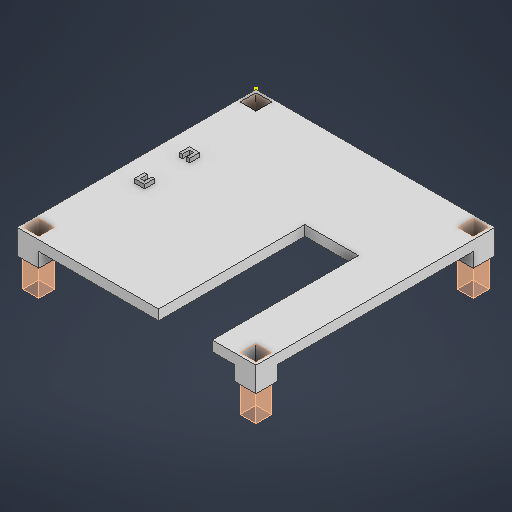
# Autodesk Inventor part: piano superiore
Saved by Autodesk Inventor 2026.2 (Build 302298000, 298)
## iProperties
Created: 2026-01-19
Part Number: piano superiore
Material: Generic
Document SubType Name: Modeling
Designer: ASUS
Density: 1 g/cm^3
Appearance: Default
Author: ASUS
Autodesk Inventor part; units mm, degrees
ref_plane "YZ Plane" through (0, 0, 0) normal (1, 0, 0) x (0, 1, 0)
ref_plane "XZ Plane" through (0, 0, 0) normal (0, 1, 0) x (-1, 0, 0)
ref_plane "XY Plane" through (0, 0, 0) normal (0, 0, 1) x (1, 0, 0)
sketch "Sketch1" plane through (0, 0, 0) normal (0, 1, 0) x (-1, 0, 0)
  line L0 (0, 0) -> (-165, 0)
  line L1 (-165, 0) -> (-165, 165)
  line L2 (-165, 165) -> (0, 165)
  line L3 (0, 165) -> (0, 0)
  line L4 (-165, 165) -> (-150, 165)
  line L5 (-165, 150) -> (-165, 165)
  line L6 (-163, 152) -> (-152, 152)
  line L7 (-152, 152) -> (-152, 163)
  line L8 (-152, 163) -> (-163, 163)
  line L9 (-163, 163) -> (-163, 152)
  line L10 (-2, 152) -> (-13, 152)
  line L11 (-13, 152) -> (-13, 163)
  line L12 (-13, 163) -> (-2, 163)
  line L13 (-2, 163) -> (-2, 152)
  line L14 (-163, 13) -> (-152, 13)
  line L15 (-152, 13) -> (-152, 2)
  line L16 (-152, 2) -> (-163, 2)
  line L17 (-163, 2) -> (-163, 13)
  line L18 (-2, 13) -> (-13, 13)
  line L19 (-13, 13) -> (-13, 2)
  line L20 (-13, 2) -> (-2, 2)
  line L21 (-2, 2) -> (-2, 13)
  line L22 (-150, 150) -> (-165, 150)
  line L23 (-165, 150) -> (-165, 165)
  line L24 (-165, 165) -> (-150, 165)
  line L25 (-150, 165) -> (-150, 150)
  line L26 (-150, 15) -> (-165, 15)
  line L27 (-165, 15) -> (-165, 0)
  line L28 (-165, 0) -> (-150, 0)
  line L29 (-150, 0) -> (-150, 15)
  line L30 (-15, 15) -> (0, 15)
  line L31 (0, 15) -> (0, 0)
  line L32 (0, 0) -> (-15, 0)
  line L33 (-15, 0) -> (-15, 15)
  line L34 (-15, 150) -> (0, 150)
  line L35 (0, 150) -> (0, 165)
  line L36 (0, 165) -> (-15, 165)
  line L37 (-15, 165) -> (-15, 150)
  line L38 (-165, 165) -> (-133.75, 165)
  line L39 (-133.75, 165) -> (-97.75, 165)
  line L40 (-97.75, 165) -> (-97.75, 64)
  line L41 (-97.75, 64) -> (-133.75, 64)
  line L42 (-133.75, 64) -> (-133.75, 165)
  point P0 (0, 15)
  dimension "d0" = 165
  dimension "d1" = 165
  dimension "d5" = 2
  dimension "d6" = 2
  dimension "d7" = 2
  dimension "d8" = 2
  dimension "d9" = 31.25
  dimension "d10" = 36
  dimension "d11" = 101
  constraints: 86 end point, 8 parallel, 4 perpendicular, 3 horizontal, 1 point on line, 13 other
  measures "d0" distance of L1.end L2.end
  measures "d1" distance of L0.end L1.end
  measures "d5" distance between parallel lines of L6 L22
  measures "d6" distance between parallel lines of L14 L26
  measures "d7" distance between parallel lines of L18 L30
  measures "d8" distance between parallel lines of L10 L34
  measures "d9" distance of L23.end L38.end
  measures "d10" distance of L40.end L41.end
  measures "d11" distance of L39.end L40.end
extrude "Extrusion1" add sketch "Sketch1" along normal blind 7 contours L0 L29 L26 L1 L22 L25 L2 L42 L41 L40 L37 L34 L3 L30 L33
sketch "Sketch2" plane through (0, 7, 0) normal (0, 1, 0) x (1, 0, 0)
  line L0 (15, -15) -> (0, -15) projected
  line L1 (15, -15) -> (0, -15)
  line L2 (0, -15) -> (0, 0)
  line L3 (0, 0) -> (15, 0)
  line L4 (15, 0) -> (15, -15)
  line L5 (150, -15) -> (150, 0) projected
  line L6 (150, -15) -> (165, -15)
  line L7 (165, -15) -> (165, 0)
  line L8 (165, 0) -> (150, 0)
  line L9 (150, 0) -> (150, -15)
  line L10 (150, -150) -> (165, -150) projected
  line L11 (150, -150) -> (165, -150)
  line L12 (165, -150) -> (165, -165)
  line L13 (165, -165) -> (150, -165)
  line L14 (150, -165) -> (150, -150)
  line L15 (15, -150) -> (0, -150)
  line L16 (0, -150) -> (0, -165)
  line L17 (0, -165) -> (15, -165)
  line L18 (15, -165) -> (15, -150)
  line L19 (2, -163) -> (2, -152)
  line L20 (2, -152) -> (13, -152)
  line L21 (13, -152) -> (13, -163)
  line L22 (13, -163) -> (2, -163)
  line L23 (2, -2) -> (2, -13)
  line L24 (2, -13) -> (13, -13)
  line L25 (13, -13) -> (13, -2)
  line L26 (13, -2) -> (2, -2)
  line L27 (163, -2) -> (163, -13)
  line L28 (163, -13) -> (152, -13)
  line L29 (152, -13) -> (152, -2)
  line L30 (152, -2) -> (163, -2)
  line L31 (163, -163) -> (163, -152)
  line L32 (163, -152) -> (152, -152)
  line L33 (152, -152) -> (152, -163)
  line L34 (152, -163) -> (163, -163)
  dimension "d14" = 15
  dimension "d15" = 15
  dimension "d16" = 15
  dimension "d17" = 15
  dimension "d18" = 15
  dimension "d19" = 15
  dimension "d20" = 15
  dimension "d21" = 15
  dimension "d22" = 2
  dimension "d23" = 2
  dimension "d24" = 2
  dimension "d25" = 2
  constraints: 64 end point, 16 parallel, 8 perpendicular, 4 horizontal, 2 point on line, 12 other
  measures "d14" distance of L2.end L3.end
  measures "d15" distance of L1.end L2.end
  measures "d16" distance of L8.end L7.end
  measures "d17" distance of L7.end L6.end
  measures "d18" distance of L12.end L13.end
  measures "d19" distance of L11.end L12.end
  measures "d20" distance of L17.end L16.end
  measures "d21" distance of L16.end L15.end
  measures "d22" distance between parallel lines of L16 L19
  measures "d23" distance between parallel lines of L2 L23
  measures "d24" distance between parallel lines of L7 L27
  measures "d25" distance between parallel lines of L12 L31
extrude "Extrusion2" add sketch "Sketch2" against normal blind 17
sketch "Sketch3" plane through (0, 7, 0) normal (0, 1, 0) x (1, 0, 0)
  point P0 (0, 0)
surface extrude "ExtrusionSrf1" sketch "Sketch2" against normal blind 37 shown yes curves L21 L22 L19 L20
surface extrude "ExtrusionSrf2" sketch "Sketch2" against normal blind 37 shown yes curves L27 L28 L29 L30
surface extrude "ExtrusionSrf3" sketch "Sketch2" against normal blind 37 shown yes curves L25 L26 L23 L24
surface extrude "ExtrusionSrf4" sketch "Sketch2" against normal blind 37 shown yes curves L31 L32 L33 L34
sketch "Sketch4" plane through (133.75, 0, 64) normal (-1, 0, 0) x (0, 0, 1)
  line L0 (0, 7) -> (101, 7) projected
  line L1 (101, 0) -> (101, 7) projected
  line L2 (0, 7) -> (101, 7)
  line L3 (101, 7) -> (101, 0)
  line L4 (101, 0) -> (0, 0)
  line L5 (0, 0) -> (0, 7)
  line L6 (0, 0) -> (0, 7) projected
  line L7 (0, 7) -> (101, 7)
  line L8 (101, 7) -> (101, 0)
  line L9 (101, 0) -> (0, 0)
  line L10 (0, 0) -> (0, 7)
  point P0 (-64, 0)
  constraints: 16 end point, 4 perpendicular, 2 horizontal, 2 parallel
extrude "Extrusion3" cut sketch "Sketch4" against normal blind 1
sketch "Sketch5" plane through (0, 7, 0) normal (0, 1, 0) x (1, 0, 0)
  line L0 (13, -2) -> (13, -13) projected
  line L1 (0, 0) -> (0, -165) projected
  line L2 (16, -67) -> (19, -67)
  line L3 (19, -67) -> (19, -62)
  line L4 (19, -62) -> (16, -62)
  line L5 (16, -62) -> (16, -67)
  line L6 (21, -60) -> (21, -67)
  line L7 (14, -67) -> (14, -60)
  line L8 (14, -60) -> (21, -60)
  line L9 (21, -67) -> (14, -67)
  line L10 (19, -90.9991) -> (19, -95.9991)
  line L11 (19, -95.9991) -> (16, -95.9991)
  line L12 (16, -95.9991) -> (16, -90.9995)
  line L13 (21, -97.9995) -> (21, -90.9991)
  line L14 (14, -90.9995) -> (14, -97.9995)
  line L15 (14, -97.9995) -> (21, -97.9995)
  line L16 (19, -90.9991) -> (19, -95.9991)
  line L17 (16, -95.9991) -> (16, -90.9995)
  line L18 (14, -90.9995) -> (14, -97.9995)
  line L19 (21, -97.9995) -> (21, -90.9991)
  line L20 (19, -67) -> (21, -67)
  line L21 (21, -60) -> (14, -60)
  line L22 (14, -67) -> (16, -67)
  line L23 (16, -62) -> (19, -62)
  line L24 (19, -90.9991) -> (21, -90.9991)
  line L25 (16, -90.9995) -> (14, -90.9995)
  line L26 (14, -97.9995) -> (16, -97.9995)
  line L27 (16, -97.9995) -> (16, -90.9995)
  line L28 (16, -90.9995) -> (14, -90.9995)
  line L29 (14, -90.9995) -> (14, -97.9995)
  line L30 (16, -97.9995) -> (21, -97.9995)
  line L31 (21, -97.9995) -> (21, -95.9991)
  line L32 (21, -95.9991) -> (16, -95.9991)
  line L33 (16, -95.9991) -> (16, -97.9995)
  line L34 (21, -90.9991) -> (19, -90.9991)
  line L35 (19, -90.9991) -> (19, -95.9991)
  line L36 (19, -95.9991) -> (21, -95.9991)
  line L37 (21, -95.9991) -> (21, -90.9991)
  line L38 (19, -67) -> (21, -67)
  line L39 (21, -67) -> (21, -60)
  line L40 (21, -60) -> (19, -60)
  line L41 (19, -60) -> (19, -67)
  line L42 (19, -60) -> (14, -60)
  line L43 (14, -60) -> (14, -62)
  line L44 (14, -62) -> (19, -62)
  line L45 (19, -62) -> (19, -60)
  line L46 (16, -62) -> (14, -62)
  line L47 (14, -62) -> (14, -67)
  line L48 (14, -67) -> (16, -67)
  line L49 (16, -67) -> (16, -62)
  dimension "d42" = 3
  dimension "d43" = 5
  dimension "d44" = 2
  constraints: 96 end point, 15 parallel, 10 horizontal, 9 perpendicular, 6 collinear, 3 point on line
  measures "d42" distance of L4.end L3.end
  measures "d43" distance of L3.end L2.end
  measures "d44" distance between parallel lines of L3 L6
extrude "Extrusion4" add sketch "Sketch5" along normal blind 2.7 contours L9 L7 L44 L5 | L3 L41 L8 L6 L9 | L44 L7 L8 L41 L4 | L24 L13 L32 L10 | L32 L13 L15 L27 L11 | L27 L15 L14 L25 L12
body "Solid1"
body "Srf1"
body "Srf2"
body "Srf3"
body "Srf4"
